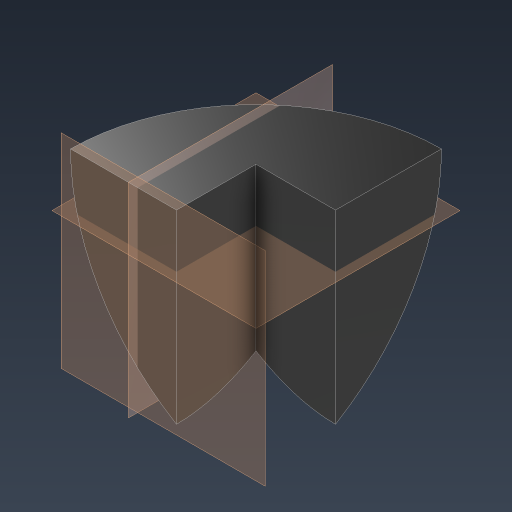
# Autodesk Inventor part: пробник
Saved by Autodesk Inventor 2023.2 (Build 272271030, 271C)
## iProperties
Created: 2025-08-20
Part Number: пробник
Material: Типовые
Document SubType Name: Modeling
Designer: Олег Коноваленко
Density: 1 g/cm^3
Appearance: Глянцевая — черная
Author: Олег Коноваленко
Autodesk Inventor part; units mm, degrees
sketch "Эскиз1" plane through (0, 0, 0) normal (0, 0, 1) x (1, 0, 0)
  line L0 (-25.3526, 20.1556) -> (14.6474, 20.1556)
  line L1 (14.6474, 20.1556) -> (14.6474, -49.8444)
  arc A0 (-25.3526, 20.1556) -> (14.6474, -49.8444) centre (55.8974, 20.1556) ccw
  line L2 (14.6474, 20.1556) -> (-14.6474, -20.1556) construction
  line L3 (44.6474, 17.5) -> (44.6474, -17.5)
  line L4 (-52.7563, 0) -> (74.0063, 0) projected
  line L5 (14.6474, -49.8444) -> (14.6474, 20.1556)
  point P0 (0, 0)
  point P1 (0, 0)
  point P2 (44.6474, 0)
  dimension "d0" = 40
  dimension "d1" = 70
  dimension "d3" = 35
  dimension "d6" = 70
  constraints: 10 end point, 3 point on circle, 2 midpoint, 1 centre point, 1 coincident, 1 horizontal, 1 line through centre, 1 perpendicular, 1 point on line, 1 vertical
  measures "d0" distance of L0.start L0.end
  measures "d1" distance of L0.end L1.end
  measures "d3" distance of L3.start L3.end
  measures "d6" distance from line of L0.start L3
revolve "Вращение1" add sketch "Эскиз1" angle 90 about axis through (44.6474, 17.5, 0) along (0, -1, 0)
sketch "Эскиз4" plane through (-25.3526, 20.1556, 0) normal (0, 1, 0) x (1, 0, 0)
  line L0 (70, 0) -> (40, 0)
  line L1 (40, 0) -> (40, 30)
  line L2 (40, 30) -> (70, 30)
  line L3 (70, 30) -> (70, 0)
  point P0 (25.3526, 0)
  point P1 (70, 30)
  point P2 (40, 0)
  dimension "d10" = 30
  constraints: 8 end point, 2 parallel, 2 perpendicular, 2 point on line, 1 horizontal
  measures "d10" distance of L1.end L2.end
extrude "Выдавливание2" cut sketch "Эскиз4" against normal up to next
